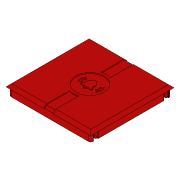
# Autodesk Inventor part: AP-03
Saved by Autodesk Inventor 2018 (Build 220112000, 112)
## iProperties
Created: 2017-11-29
Part Number: AP-03
Material: Q235
Document SubType Name: Modeling
Designer: Lars von Hebel
Mass: 170.489 g
Surface Area: 186.324 cm^2
Volume: 21.7183 cm^3
Density: 7.85 g/cm^3
Appearance: Red
RuleStatus: InUse
Author: Lars von Hebel
Autodesk Inventor part; units mm, degrees
(part 1 of 2)
ref_plane "YZ Plane" through (0, 0, 0) normal (1, 0, 0) x (0, 1, 0)
sketch "Block1" plane through (0, 0, 0) normal (0, 0, 1) x (1, 0, 0)
  spline S0 degree 3 poles (131.0781, -293.1362) (132.5466, -291.7994) (133.2816, -290.1204) (133.2816, -288.0985) (133.2816, -286.1085) (132.5466, -284.4599) (131.0781, -283.1542) knots 0 0 0 0 1 1 1 2 2 2 2
  line L0 (131.0781, -293.1362) -> (132.5466, -291.7994) construction
  line L1 (132.5466, -291.7994) -> (133.2816, -290.1204) construction
  line L2 (133.2816, -290.1204) -> (133.2816, -288.0985) construction
  line L3 (133.2816, -288.0985) -> (133.2816, -286.1085) construction
  line L4 (133.2816, -286.1085) -> (132.5466, -284.4599) construction
  line L5 (132.5466, -284.4599) -> (131.0781, -283.1542) construction
  spline S1 degree 3 poles (131.0781, -283.1542) (129.6082, -281.8485) (127.5611, -281.1953) (124.9359, -281.1953) knots 2 2 2 2 3 3 3 3
  line L6 (131.0781, -283.1542) -> (129.6082, -281.8485) construction
  line L7 (129.6082, -281.8485) -> (127.5611, -281.1953) construction
  line L8 (127.5611, -281.1953) -> (124.9359, -281.1953) construction
  line L9 (124.9359, -281.1953) -> (116.4022, -281.1953)
  line L10 (116.4022, -281.1953) -> (116.4022, -295.1414)
  line L11 (116.4022, -295.1414) -> (124.9359, -295.1414)
  spline S2 degree 3 poles (124.9359, -295.1414) (127.5611, -295.1414) (129.6082, -294.473) (131.0781, -293.1362) knots 6 6 6 6 7 7 7 7
  line L12 (124.9359, -295.1414) -> (127.5611, -295.1414) construction
  line L13 (127.5611, -295.1414) -> (129.6082, -294.473) construction
  line L14 (129.6082, -294.473) -> (131.0781, -293.1362) construction
  spline S3 degree 3 poles (135.1103, -309.0643) (133.2967, -307.7434) (130.8741, -307.0822) (127.8425, -307.0822) knots 0 0 0 0 1 1 1 1
  line L15 (135.1103, -309.0643) -> (133.2967, -307.7434) construction
  line L16 (133.2967, -307.7434) -> (130.8741, -307.0822) construction
  line L17 (130.8741, -307.0822) -> (127.8425, -307.0822) construction
  line L18 (127.8425, -307.0822) -> (116.4022, -307.0822)
  line L19 (116.4022, -307.0822) -> (116.4022, -322.4743)
  line L20 (116.4022, -322.4743) -> (125.592, -322.4743)
  spline S4 degree 3 poles (125.592, -322.4743) (129.9366, -322.4743) (133.0624, -321.876) (134.9699, -320.6788) knots 4 4 4 4 5 5 5 5
  line L21 (125.592, -322.4743) -> (129.9366, -322.4743) construction
  line L22 (129.9366, -322.4743) -> (133.0624, -321.876) construction
  line L23 (133.0624, -321.876) -> (134.9699, -320.6788) construction
  spline S5 degree 3 poles (134.9699, -320.6788) (136.876, -319.4816) (137.8294, -317.4063) (137.8294, -314.452) (137.8294, -312.182) (136.923, -310.3866) (135.1103, -309.0643) knots 5 5 5 5 6 6 6 7 7 7 7
  line L24 (134.9699, -320.6788) -> (136.876, -319.4816) construction
  line L25 (136.876, -319.4816) -> (137.8294, -317.4063) construction
  line L26 (137.8294, -317.4063) -> (137.8294, -314.452) construction
  line L27 (137.8294, -314.452) -> (137.8294, -312.182) construction
  line L28 (137.8294, -312.182) -> (136.923, -310.3866) construction
  line L29 (136.923, -310.3866) -> (135.1103, -309.0643) construction
  spline S6 degree 3 poles (123.151, -216.2055) (123.151, -206.5504) (130.9712, -198.7334) (140.6263, -198.7334) knots 0 0 0 0 1 1 1 1
  line L30 (123.151, -216.2055) -> (123.151, -206.5504) construction
  line L31 (123.151, -206.5504) -> (130.9712, -198.7334) construction
  line L32 (130.9712, -198.7334) -> (140.6263, -198.7334) construction
  line L33 (140.6263, -198.7334) -> (140.6263, -159.7323)
  spline S7 degree 3 poles (140.6263, -159.7323) (140.6263, -132.2619) (159.7288, -109.3026) (185.3549, -103.2715) knots 2 2 2 2 3 3 3 3
  line L34 (140.6263, -159.7323) -> (140.6263, -132.2619) construction
  line L35 (140.6263, -132.2619) -> (159.7288, -109.3026) construction
  line L36 (159.7288, -109.3026) -> (185.3549, -103.2715) construction
  spline S8 degree 3 poles (185.3549, -103.2715) (185.5067, -96.0755) (191.4085, -90.2514) (198.6594, -90.2514) (205.9045, -90.2514) (211.78, -96.0498) (211.9356, -103.2715) knots 3 3 3 3 4 4 4 5 5 5 5
  line L37 (185.3549, -103.2715) -> (185.5067, -96.0755) construction
  line L38 (185.5067, -96.0755) -> (191.4085, -90.2514) construction
  line L39 (191.4085, -90.2514) -> (198.6594, -90.2514) construction
  line L40 (198.6594, -90.2514) -> (205.9045, -90.2514) construction
  line L41 (205.9045, -90.2514) -> (211.78, -96.0498) construction
  line L42 (211.78, -96.0498) -> (211.9356, -103.2715) construction
  spline S9 degree 3 poles (211.9356, -103.2715) (237.5617, -109.3026) (256.6634, -132.2619) (256.6634, -159.7323) knots 5 5 5 5 6 6 6 6
  line L43 (211.9356, -103.2715) -> (237.5617, -109.3026) construction
  line L44 (237.5617, -109.3026) -> (256.6634, -132.2619) construction
  line L45 (256.6634, -132.2619) -> (256.6634, -159.7323) construction
  line L46 (256.6634, -159.7323) -> (256.6634, -198.7334)
  spline S10 degree 3 poles (256.6634, -198.7334) (266.3194, -198.7334) (274.1356, -206.5504) (274.1356, -216.2055) knots 7 7 7 7 8 8 8 8
  line L47 (256.6634, -198.7334) -> (266.3194, -198.7334) construction
  line L48 (266.3194, -198.7334) -> (274.1356, -206.5504) construction
  line L49 (274.1356, -206.5504) -> (274.1356, -216.2055) construction
  line L50 (274.1356, -216.2055) -> (274.1356, -228.533)
  line L51 (274.1356, -228.533) -> (123.151, -228.533)
  line L52 (123.151, -228.533) -> (123.151, -216.2055)
  spline S11 degree 3 poles (75.656, -215.1488) (74.5193, -215.883) (73.2455, -216.2339) (71.9859, -216.2339) (69.7638, -216.2339) (67.5867, -215.1414) (66.2906, -213.1359) (55.8364, -196.9575) (50.3107, -178.1799) (50.3107, -158.8331) (50.3107, -139.9897) (55.5725, -121.6274) (65.5276, -105.7302) (67.5128, -102.5603) (71.6917, -101.5976) (74.8633, -103.5844) (78.0341, -105.57) (78.9947, -109.7497) (77.0092, -112.92) (68.4053, -126.6596) (63.8576, -142.536) (63.8576, -158.8331) (63.8576, -175.5656) (68.6335, -191.8008) (77.6688, -205.7835) (79.699, -208.9255) (78.7979, -213.1184) (75.656, -215.1488) knots 0 0 0 0 1 1 1 2 2 2 3 3 3 4 4 4 5 5 5 6 6 6 7 7 7 8 8 8 9 9 9 9
  line L53 (75.656, -215.1488) -> (74.5193, -215.883) construction
  line L54 (74.5193, -215.883) -> (73.2455, -216.2339) construction
  line L55 (73.2455, -216.2339) -> (71.9859, -216.2339) construction
  line L56 (71.9859, -216.2339) -> (69.7638, -216.2339) construction
  line L57 (69.7638, -216.2339) -> (67.5867, -215.1414) construction
  line L58 (67.5867, -215.1414) -> (66.2906, -213.1359) construction
  line L59 (66.2906, -213.1359) -> (55.8364, -196.9575) construction
  line L60 (55.8364, -196.9575) -> (50.3107, -178.1799) construction
  line L61 (50.3107, -178.1799) -> (50.3107, -158.8331) construction
  line L62 (50.3107, -158.8331) -> (50.3107, -139.9897) construction
  line L63 (50.3107, -139.9897) -> (55.5725, -121.6274) construction
  line L64 (55.5725, -121.6274) -> (65.5276, -105.7302) construction
  line L65 (65.5276, -105.7302) -> (67.5128, -102.5603) construction
  line L66 (67.5128, -102.5603) -> (71.6917, -101.5976) construction
  line L67 (71.6917, -101.5976) -> (74.8633, -103.5844) construction
  line L68 (74.8633, -103.5844) -> (78.0341, -105.57) construction
  line L69 (78.0341, -105.57) -> (78.9947, -109.7497) construction
  line L70 (78.9947, -109.7497) -> (77.0092, -112.92) construction
  line L71 (77.0092, -112.92) -> (68.4053, -126.6596) construction
  line L72 (68.4053, -126.6596) -> (63.8576, -142.536) construction
  line L73 (63.8576, -142.536) -> (63.8576, -158.8331) construction
  line L74 (63.8576, -158.8331) -> (63.8576, -175.5656) construction
  line L75 (63.8576, -175.5656) -> (68.6335, -191.8008) construction
  line L76 (68.6335, -191.8008) -> (77.6688, -205.7835) construction
  line L77 (77.6688, -205.7835) -> (79.699, -208.9255) construction
  line L78 (79.699, -208.9255) -> (78.7979, -213.1184) construction
  line L79 (78.7979, -213.1184) -> (75.656, -215.1488) construction
  spline S12 degree 3 poles (91.7394, -196.7237) (84.4441, -185.4332) (80.5881, -172.331) (80.5881, -158.8331) (80.5881, -145.6846) (84.2605, -132.8708) (91.2083, -121.7772) (93.0767, -118.7927) (97.0101, -117.8885) (99.9949, -119.7577) (102.9789, -121.6266) (103.8828, -125.5604) (102.0143, -128.5443) (96.3382, -137.6073) (93.3382, -148.0811) (93.3382, -158.8331) (93.3382, -169.8707) (96.4884, -180.5803) (102.4482, -189.804) (104.359, -192.7611) (103.5109, -196.7078) (100.5536, -198.6182) (99.484, -199.3093) (98.2848, -199.6396) (97.0996, -199.6396) (95.0078, -199.6396) (92.9592, -198.6112) (91.7394, -196.7237) knots 0 0 0 0 1 1 1 2 2 2 3 3 3 4 4 4 5 5 5 6 6 6 7 7 7 8 8 8 9 9 9 9
  line L80 (91.7394, -196.7237) -> (84.4441, -185.4332) construction
  line L81 (84.4441, -185.4332) -> (80.5881, -172.331) construction
  line L82 (80.5881, -172.331) -> (80.5881, -158.8331) construction
  line L83 (80.5881, -158.8331) -> (80.5881, -145.6846) construction
  line L84 (80.5881, -145.6846) -> (84.2605, -132.8708) construction
  line L85 (84.2605, -132.8708) -> (91.2083, -121.7772) construction
  line L86 (91.2083, -121.7772) -> (93.0767, -118.7927) construction
  line L87 (93.0767, -118.7927) -> (97.0101, -117.8885) construction
  line L88 (97.0101, -117.8885) -> (99.9949, -119.7577) construction
  line L89 (99.9949, -119.7577) -> (102.9789, -121.6266) construction
  line L90 (102.9789, -121.6266) -> (103.8828, -125.5604) construction
  line L91 (103.8828, -125.5604) -> (102.0143, -128.5443) construction
  line L92 (102.0143, -128.5443) -> (96.3382, -137.6073) construction
  line L93 (96.3382, -137.6073) -> (93.3382, -148.0811) construction
  line L94 (93.3382, -148.0811) -> (93.3382, -158.8331) construction
  line L95 (93.3382, -158.8331) -> (93.3382, -169.8707) construction
  line L96 (93.3382, -169.8707) -> (96.4884, -180.5803) construction
  line L97 (96.4884, -180.5803) -> (102.4482, -189.804) construction
  line L98 (102.4482, -189.804) -> (104.359, -192.7611) construction
  line L99 (104.359, -192.7611) -> (103.5109, -196.7078) construction
  line L100 (103.5109, -196.7078) -> (100.5536, -198.6182) construction
  line L101 (100.5536, -198.6182) -> (99.484, -199.3093) construction
  line L102 (99.484, -199.3093) -> (98.2848, -199.6396) construction
  line L103 (98.2848, -199.6396) -> (97.0996, -199.6396) construction
  line L104 (97.0996, -199.6396) -> (95.0078, -199.6396) construction
  line L105 (95.0078, -199.6396) -> (92.9592, -198.6112) construction
  line L106 (92.9592, -198.6112) -> (91.7394, -196.7237) construction
  spline S13 degree 3 poles (149.2234, -329.0939) (145.3157, -332.6421) (139.5648, -334.4151) (131.9686, -334.4151) knots 0 0 0 0 1 1 1 1
  line L107 (149.2234, -329.0939) -> (145.3157, -332.6421) construction
  line L108 (145.3157, -332.6421) -> (139.5648, -334.4151) construction
  line L109 (139.5648, -334.4151) -> (131.9686, -334.4151) construction
  line L110 (131.9686, -334.4151) -> (100.0857, -334.4151)
  line L111 (100.0857, -334.4151) -> (100.0857, -269.2545)
  line L112 (100.0857, -269.2545) -> (128.4053, -269.2545)
  spline S14 degree 3 poles (128.4053, -269.2545) (135.1573, -269.2545) (140.4625, -270.8705) (144.3239, -274.1019) knots 4 4 4 4 5 5 5 5
  line L113 (128.4053, -269.2545) -> (135.1573, -269.2545) construction
  line L114 (135.1573, -269.2545) -> (140.4625, -270.8705) construction
  line L115 (140.4625, -270.8705) -> (144.3239, -274.1019) construction
  spline S15 degree 3 poles (144.3239, -274.1019) (148.1839, -277.3332) (150.1146, -281.1548) (150.1146, -285.5667) (150.1146, -291.2221) (147.1292, -295.5566) (141.1584, -298.5702) knots 5 5 5 5 6 6 6 7 7 7 7
  line L116 (144.3239, -274.1019) -> (148.1839, -277.3332) construction
  line L117 (148.1839, -277.3332) -> (150.1146, -281.1548) construction
  line L118 (150.1146, -281.1548) -> (150.1146, -285.5667) construction
  line L119 (150.1146, -285.5667) -> (150.1146, -291.2221) construction
  line L120 (150.1146, -291.2221) -> (147.1292, -295.5566) construction
  line L121 (147.1292, -295.5566) -> (141.1584, -298.5702) construction
  spline S16 degree 3 poles (141.1584, -298.5702) (145.66, -299.7529) (149.1062, -301.8377) (151.4977, -304.8245) knots 7 7 7 7 8 8 8 8
  line L122 (141.1584, -298.5702) -> (145.66, -299.7529) construction
  line L123 (145.66, -299.7529) -> (149.1062, -301.8377) construction
  line L124 (149.1062, -301.8377) -> (151.4977, -304.8245) construction
  spline S17 degree 3 poles (151.4977, -304.8245) (153.8885, -307.8121) (155.0842, -311.2966) (155.0842, -315.2788) (155.0842, -320.9421) (153.1304, -325.5472) (149.2234, -329.0939) knots 8 8 8 8 9 9 9 10 10 10 10
  line L125 (151.4977, -304.8245) -> (153.8885, -307.8121) construction
  line L126 (153.8885, -307.8121) -> (155.0842, -311.2966) construction
  line L127 (155.0842, -311.2966) -> (155.0842, -315.2788) construction
  line L128 (155.0842, -315.2788) -> (155.0842, -320.9421) construction
  line L129 (155.0842, -320.9421) -> (153.1304, -325.5472) construction
  line L130 (153.1304, -325.5472) -> (149.2234, -329.0939) construction
  line L131 (210.0365, -334.4151) -> (196.1114, -334.4151)
  line L132 (196.1114, -334.4151) -> (196.1114, -328.1181)
  spline S18 degree 3 poles (196.1114, -328.1181) (192.0156, -332.8757) (187.2493, -335.2549) (181.8102, -335.2549) (176.9961, -335.2549) (173.0891, -333.7778) (170.0886, -330.8235) knots 2 2 2 2 3 3 3 4 4 4 4
  line L133 (196.1114, -328.1181) -> (192.0156, -332.8757) construction
  line L134 (192.0156, -332.8757) -> (187.2493, -335.2549) construction
  line L135 (187.2493, -335.2549) -> (181.8102, -335.2549) construction
  line L136 (181.8102, -335.2549) -> (176.9961, -335.2549) construction
  line L137 (176.9961, -335.2549) -> (173.0891, -333.7778) construction
  line L138 (173.0891, -333.7778) -> (170.0886, -330.8235) construction
  spline S19 degree 3 poles (170.0886, -330.8235) (167.088, -327.87) (165.5877, -323.7807) (165.5877, -318.5564) knots 4 4 4 4 5 5 5 5
  line L139 (170.0886, -330.8235) -> (167.088, -327.87) construction
  line L140 (167.088, -327.87) -> (165.5877, -323.7807) construction
  line L141 (165.5877, -323.7807) -> (165.5877, -318.5564) construction
  line L142 (165.5877, -318.5564) -> (165.5877, -290.3837)
  line L143 (165.5877, -290.3837) -> (179.5127, -290.3837)
  line L144 (179.5127, -290.3837) -> (179.5127, -317.5878)
  spline S20 degree 3 poles (179.5127, -317.5878) (179.5127, -323.1774) (181.8413, -325.9725) (186.4991, -325.9725) (189.125, -325.9725) (191.3675, -324.9562) (193.2273, -322.922) (195.0871, -320.8879) (196.0174, -319.3898) (196.0174, -318.427) knots 8 8 8 8 9 9 9 10 10 10 11 11 11 11
  line L145 (179.5127, -317.5878) -> (179.5127, -323.1774) construction
  line L146 (179.5127, -323.1774) -> (181.8413, -325.9725) construction
  line L147 (181.8413, -325.9725) -> (186.4991, -325.9725) construction
  line L148 (186.4991, -325.9725) -> (189.125, -325.9725) construction
  line L149 (189.125, -325.9725) -> (191.3675, -324.9562) construction
  line L150 (191.3675, -324.9562) -> (193.2273, -322.922) construction
  line L151 (193.2273, -322.922) -> (195.0871, -320.8879) construction
  line L152 (195.0871, -320.8879) -> (196.0174, -319.3898) construction
  line L153 (196.0174, -319.3898) -> (196.0174, -318.427) construction
  line L154 (196.0174, -318.427) -> (196.0174, -290.3837)
  line L155 (196.0174, -290.3837) -> (210.0365, -290.3837)
  line L156 (210.0365, -290.3837) -> (210.0365, -334.4151)
  spline S21 degree 3 poles (198.6594, -257.2646) (187.0631, -257.2646) (177.3823, -249.4732) (174.3278, -238.8543) knots 0 0 0 0 1 1 1 1
  line L157 (198.6594, -257.2646) -> (187.0631, -257.2646) construction
  line L158 (187.0631, -257.2646) -> (177.3823, -249.4732) construction
  line L159 (177.3823, -249.4732) -> (174.3278, -238.8543) construction
  line L160 (174.3278, -238.8543) -> (222.9549, -238.8543)
  spline S22 degree 3 poles (222.9549, -238.8543) (219.9074, -249.4732) (210.2266, -257.2646) (198.6594, -257.2646) knots 2 2 2 2 3 3 3 3
  line L161 (222.9549, -238.8543) -> (219.9074, -249.4732) construction
  line L162 (219.9074, -249.4732) -> (210.2266, -257.2646) construction
  line L163 (210.2266, -257.2646) -> (198.6594, -257.2646) construction
  line L164 (263.066, -324.9468) -> (263.066, -334.4151)
  line L165 (263.066, -334.4151) -> (217.632, -334.4151)
  line L166 (217.632, -334.4151) -> (240.3605, -299.8527)
  line L167 (240.3605, -299.8527) -> (219.8354, -299.8527)
  line L168 (219.8354, -299.8527) -> (219.8354, -290.3837)
  line L169 (219.8354, -290.3837) -> (263.066, -290.3837)
  line L170 (263.066, -290.3837) -> (240.3924, -324.9468)
  line L171 (240.3924, -324.9468) -> (263.066, -324.9468)
  line L172 (313.0949, -324.9468) -> (313.0949, -334.4151)
  line L173 (313.0949, -334.4151) -> (267.6609, -334.4151)
  line L174 (267.6609, -334.4151) -> (290.3895, -299.8527)
  line L175 (290.3895, -299.8527) -> (269.8643, -299.8527)
  line L176 (269.8643, -299.8527) -> (269.8643, -290.3837)
  line L177 (269.8643, -290.3837) -> (313.0949, -290.3837)
  line L178 (313.0949, -290.3837) -> (290.4213, -324.9468)
  line L179 (290.4213, -324.9468) -> (313.0949, -324.9468)
  spline S23 degree 3 poles (307.939, -196.7233) (306.7188, -198.6108) (304.6691, -199.6396) (302.5773, -199.6396) (301.3928, -199.6396) (300.1944, -199.3097) (299.1251, -198.6187) (296.1664, -196.7078) (295.3182, -192.7615) (297.2295, -189.8043) (303.1889, -180.5799) (306.3391, -169.8703) (306.3391, -158.8331) (306.3391, -148.0799) (303.3383, -137.6065) (297.6622, -128.5448) (295.7944, -125.5607) (296.6972, -121.6269) (299.6808, -119.7582) (302.6644, -117.8881) (306.599, -118.7927) (308.4682, -121.7767) (315.416, -132.8692) (319.0891, -145.6835) (319.0891, -158.8331) (319.0891, -172.3302) (315.2323, -185.4328) (307.939, -196.7233) knots 0 0 0 0 1 1 1 2 2 2 3 3 3 4 4 4 5 5 5 6 6 6 7 7 7 8 8 8 9 9 9 9
  line L180 (307.939, -196.7233) -> (306.7188, -198.6108) construction
  line L181 (306.7188, -198.6108) -> (304.6691, -199.6396) construction
  line L182 (304.6691, -199.6396) -> (302.5773, -199.6396) construction
  line L183 (302.5773, -199.6396) -> (301.3928, -199.6396) construction
  line L184 (301.3928, -199.6396) -> (300.1944, -199.3097) construction
  line L185 (300.1944, -199.3097) -> (299.1251, -198.6187) construction
  line L186 (299.1251, -198.6187) -> (296.1664, -196.7078) construction
  line L187 (296.1664, -196.7078) -> (295.3182, -192.7615) construction
  line L188 (295.3182, -192.7615) -> (297.2295, -189.8043) construction
  line L189 (297.2295, -189.8043) -> (303.1889, -180.5799) construction
  line L190 (303.1889, -180.5799) -> (306.3391, -169.8703) construction
  line L191 (306.3391, -169.8703) -> (306.3391, -158.8331) construction
  line L192 (306.3391, -158.8331) -> (306.3391, -148.0799) construction
  line L193 (306.3391, -148.0799) -> (303.3383, -137.6065) construction
  line L194 (303.3383, -137.6065) -> (297.6622, -128.5448) construction
  line L195 (297.6622, -128.5448) -> (295.7944, -125.5607) construction
  line L196 (295.7944, -125.5607) -> (296.6972, -121.6269) construction
  line L197 (296.6972, -121.6269) -> (299.6808, -119.7582) construction
  line L198 (299.6808, -119.7582) -> (302.6644, -117.8881) construction
  line L199 (302.6644, -117.8881) -> (306.599, -118.7927) construction
  line L200 (306.599, -118.7927) -> (308.4682, -121.7767) construction
  line L201 (308.4682, -121.7767) -> (315.416, -132.8692) construction
  line L202 (315.416, -132.8692) -> (319.0891, -145.6835) construction
  line L203 (319.0891, -145.6835) -> (319.0891, -158.8331) construction
  line L204 (319.0891, -158.8331) -> (319.0891, -172.3302) construction
  line L205 (319.0891, -172.3302) -> (315.2323, -185.4328) construction
  line L206 (315.2323, -185.4328) -> (307.939, -196.7233) construction
  spline S24 degree 3 poles (333.3863, -213.1359) (332.0897, -215.1414) (329.9123, -216.2339) (327.6914, -216.2339) (326.4307, -216.2339) (325.1576, -215.8834) (324.0213, -215.1488) (320.879, -213.1184) (319.9778, -208.9255) (322.0074, -205.7835) (331.0438, -191.8) (335.8204, -175.5648) (335.8204, -158.8331) (335.8204, -142.5372) (331.2726, -126.6604) (322.6689, -112.92) (320.6829, -109.7493) (321.6431, -105.5696) (324.8151, -103.5844) (327.984, -101.5992) (332.1645, -102.5598) (334.1504, -105.7302) (344.1051, -121.6285) (349.3674, -139.9914) (349.3674, -158.8331) (349.3674, -178.1792) (343.8405, -196.9568) (333.3863, -213.1359) knots 0 0 0 0 1 1 1 2 2 2 3 3 3 4 4 4 5 5 5 6 6 6 7 7 7 8 8 8 9 9 9 9
  line L207 (333.3863, -213.1359) -> (332.0897, -215.1414) construction
  line L208 (332.0897, -215.1414) -> (329.9123, -216.2339) construction
  line L209 (329.9123, -216.2339) -> (327.6914, -216.2339) construction
  line L210 (327.6914, -216.2339) -> (326.4307, -216.2339) construction
  line L211 (326.4307, -216.2339) -> (325.1576, -215.8834) construction
  line L212 (325.1576, -215.8834) -> (324.0213, -215.1488) construction
  line L213 (324.0213, -215.1488) -> (320.879, -213.1184) construction
  line L214 (320.879, -213.1184) -> (319.9778, -208.9255) construction
  line L215 (319.9778, -208.9255) -> (322.0074, -205.7835) construction
  line L216 (322.0074, -205.7835) -> (331.0438, -191.8) construction
  line L217 (331.0438, -191.8) -> (335.8204, -175.5648) construction
  line L218 (335.8204, -175.5648) -> (335.8204, -158.8331) construction
  line L219 (335.8204, -158.8331) -> (335.8204, -142.5372) construction
  line L220 (335.8204, -142.5372) -> (331.2726, -126.6604) construction
  line L221 (331.2726, -126.6604) -> (322.6689, -112.92) construction
  line L222 (322.6689, -112.92) -> (320.6829, -109.7493) construction
  line L223 (320.6829, -109.7493) -> (321.6431, -105.5696) construction
  line L224 (321.6431, -105.5696) -> (324.8151, -103.5844) construction
  line L225 (324.8151, -103.5844) -> (327.984, -101.5992) construction
  line L226 (327.984, -101.5992) -> (332.1645, -102.5598) construction
  line L227 (332.1645, -102.5598) -> (334.1504, -105.7302) construction
  line L228 (334.1504, -105.7302) -> (344.1051, -121.6285) construction
  line L229 (344.1051, -121.6285) -> (349.3674, -139.9914) construction
  line L230 (349.3674, -139.9914) -> (349.3674, -158.8331) construction
  line L231 (349.3674, -158.8331) -> (349.3674, -178.1792) construction
  line L232 (349.3674, -178.1792) -> (343.8405, -196.9568) construction
  line L233 (343.8405, -196.9568) -> (333.3863, -213.1359) construction
  point P0 (186.8523, -231.4778)
sketch "Block2" plane through (0, 0, 0) normal (0, 0, 1) x (1, 0, 0)
  spline S0 degree 3 poles (199.9867, -151.4497) (199.9867, -151.7851) (200.1264, -151.9528) (200.4058, -151.9528) (200.5634, -151.9528) (200.6979, -151.8918) (200.8095, -151.7698) (200.9211, -151.6477) (200.9769, -151.5579) (200.9769, -151.5001) knots 8 8 8 8 9 9 9 10 10 10 11 11 11 11
  line L0 (199.9867, -151.4497) -> (199.9867, -151.7851) construction
  line L1 (199.9867, -151.7851) -> (200.1264, -151.9528) construction
  line L2 (200.1264, -151.9528) -> (200.4058, -151.9528) construction
  line L3 (200.4058, -151.9528) -> (200.5634, -151.9528) construction
  line L4 (200.5634, -151.9528) -> (200.6979, -151.8918) construction
  line L5 (200.6979, -151.8918) -> (200.8095, -151.7698) construction
  line L6 (200.8095, -151.7698) -> (200.9211, -151.6477) construction
  line L7 (200.9211, -151.6477) -> (200.9769, -151.5579) construction
  line L8 (200.9769, -151.5579) -> (200.9769, -151.5001) construction
  line L9 (200.9769, -151.5001) -> (200.9769, -149.8175)
  line L10 (200.9769, -149.8175) -> (201.8181, -149.8175)
  line L11 (201.8181, -149.8175) -> (201.8181, -152.4594)
  spline S1 degree 3 poles (201.1355, -147.8304) (200.4397, -147.8304) (199.8588, -147.3629) (199.6756, -146.7257) knots 0 0 0 0 1 1 1 1
  line L12 (201.1355, -147.8304) -> (200.4397, -147.8304) construction
  line L13 (200.4397, -147.8304) -> (199.8588, -147.3629) construction
  line L14 (199.8588, -147.3629) -> (199.6756, -146.7257) construction
  line L15 (199.6756, -146.7257) -> (202.5932, -146.7257)
  spline S2 degree 3 poles (202.5932, -146.7257) (202.4103, -147.3629) (201.8295, -147.8304) (201.1355, -147.8304) knots 2 2 2 2 3 3 3 3
  line L16 (202.5932, -146.7257) -> (202.4103, -147.3629) construction
  line L17 (202.4103, -147.3629) -> (201.8295, -147.8304) construction
  line L18 (201.8295, -147.8304) -> (201.1355, -147.8304) construction
  line L19 (204.9999, -151.8913) -> (204.9999, -152.4594)
  line L20 (204.9999, -152.4594) -> (202.2738, -152.4594)
  line L21 (202.2738, -152.4594) -> (203.6375, -150.3856)
  line L22 (203.6375, -150.3856) -> (202.406, -150.3856)
  line L23 (202.406, -150.3856) -> (202.406, -149.8175)
  line L24 (202.406, -149.8175) -> (204.9999, -149.8175)
  line L25 (204.9999, -149.8175) -> (203.6394, -151.8913)
  line L26 (203.6394, -151.8913) -> (204.9999, -151.8913)
  line L27 (208.0016, -151.8913) -> (208.0016, -152.4594)
  line L28 (208.0016, -152.4594) -> (205.2755, -152.4594)
  line L29 (205.2755, -152.4594) -> (206.6393, -150.3856)
  line L30 (206.6393, -150.3856) -> (205.4078, -150.3856)
  line L31 (205.4078, -150.3856) -> (205.4078, -149.8175)
  line L32 (205.4078, -149.8175) -> (208.0016, -149.8175)
  line L33 (208.0016, -149.8175) -> (206.6412, -151.8913)
  line L34 (206.6412, -151.8913) -> (208.0016, -151.8913)
  spline S3 degree 3 poles (207.6922, -144.1979) (207.619, -144.3111) (207.496, -144.3729) (207.3705, -144.3729) (207.2995, -144.3729) (207.2276, -144.3531) (207.1634, -144.3116) (206.9859, -144.1969) (206.935, -143.9602) (207.0497, -143.7827) (207.4072, -143.2293) (207.5962, -142.5867) (207.5962, -141.9245) (207.5962, -141.2793) (207.4162, -140.6509) (207.0756, -140.1072) (206.9636, -139.9281) (207.0177, -139.6921) (207.1967, -139.58) (207.3758, -139.4678) (207.6118, -139.522) (207.724, -139.7011) (208.1409, -140.3666) (208.3612, -141.1355) (208.3612, -141.9245) (208.3612, -142.7343) (208.1298, -143.5204) (207.6922, -144.1979) knots 0 0 0 0 1 1 1 2 2 2 3 3 3 4 4 4 5 5 5 6 6 6 7 7 7 8 8 8 9 9 9 9
  line L35 (207.6922, -144.1979) -> (207.619, -144.3111) construction
  line L36 (207.619, -144.3111) -> (207.496, -144.3729) construction
  line L37 (207.496, -144.3729) -> (207.3705, -144.3729) construction
  line L38 (207.3705, -144.3729) -> (207.2995, -144.3729) construction
  line L39 (207.2995, -144.3729) -> (207.2276, -144.3531) construction
  line L40 (207.2276, -144.3531) -> (207.1634, -144.3116) construction
  line L41 (207.1634, -144.3116) -> (206.9859, -144.1969) construction
  line L42 (206.9859, -144.1969) -> (206.935, -143.9602) construction
  line L43 (206.935, -143.9602) -> (207.0497, -143.7827) construction
  line L44 (207.0497, -143.7827) -> (207.4072, -143.2293) construction
  line L45 (207.4072, -143.2293) -> (207.5962, -142.5867) construction
  line L46 (207.5962, -142.5867) -> (207.5962, -141.9245) construction
  line L47 (207.5962, -141.9245) -> (207.5962, -141.2793) construction
  line L48 (207.5962, -141.2793) -> (207.4162, -140.6509) construction
  line L49 (207.4162, -140.6509) -> (207.0756, -140.1072) construction
  line L50 (207.0756, -140.1072) -> (206.9636, -139.9281) construction
  line L51 (206.9636, -139.9281) -> (207.0177, -139.6921) construction
  line L52 (207.0177, -139.6921) -> (207.1967, -139.58) construction
  line L53 (207.1967, -139.58) -> (207.3758, -139.4678) construction
  line L54 (207.3758, -139.4678) -> (207.6118, -139.522) construction
  line L55 (207.6118, -139.522) -> (207.724, -139.7011) construction
  line L56 (207.724, -139.7011) -> (208.1409, -140.3666) construction
  line L57 (208.1409, -140.3666) -> (208.3612, -141.1355) construction
  line L58 (208.3612, -141.1355) -> (208.3612, -141.9245) construction
  line L59 (208.3612, -141.9245) -> (208.3612, -142.7343) construction
  line L60 (208.3612, -142.7343) -> (208.1298, -143.5204) construction
  line L61 (208.1298, -143.5204) -> (207.6922, -144.1979) construction
  spline S4 degree 3 poles (209.2191, -145.1826) (209.1413, -145.303) (209.0106, -145.3685) (208.8774, -145.3685) (208.8017, -145.3685) (208.7253, -145.3475) (208.6572, -145.3034) (208.4686, -145.1816) (208.4146, -144.93) (208.5363, -144.7415) (209.0785, -143.9025) (209.3651, -142.9284) (209.3651, -141.9245) (209.3651, -140.9467) (209.0923, -139.9941) (208.576, -139.1697) (208.4569, -138.9794) (208.5145, -138.7287) (208.7048, -138.6095) (208.8949, -138.4904) (209.1458, -138.5481) (209.2649, -138.7383) (209.8622, -139.6922) (210.1779, -140.794) (210.1779, -141.9245) (210.1779, -143.0852) (209.8463, -144.2119) (209.2191, -145.1826) knots 0 0 0 0 1 1 1 2 2 2 3 3 3 4 4 4 5 5 5 6 6 6 7 7 7 8 8 8 9 9 9 9
  line L62 (209.2191, -145.1826) -> (209.1413, -145.303) construction
  line L63 (209.1413, -145.303) -> (209.0106, -145.3685) construction
  line L64 (209.0106, -145.3685) -> (208.8774, -145.3685) construction
  line L65 (208.8774, -145.3685) -> (208.8017, -145.3685) construction
  line L66 (208.8017, -145.3685) -> (208.7253, -145.3475) construction
  line L67 (208.7253, -145.3475) -> (208.6572, -145.3034) construction
  line L68 (208.6572, -145.3034) -> (208.4686, -145.1816) construction
  line L69 (208.4686, -145.1816) -> (208.4146, -144.93) construction
  line L70 (208.4146, -144.93) -> (208.5363, -144.7415) construction
  line L71 (208.5363, -144.7415) -> (209.0785, -143.9025) construction
  line L72 (209.0785, -143.9025) -> (209.3651, -142.9284) construction
  line L73 (209.3651, -142.9284) -> (209.3651, -141.9245) construction
  line L74 (209.3651, -141.9245) -> (209.3651, -140.9467) construction
  line L75 (209.3651, -140.9467) -> (209.0923, -139.9941) construction
  line L76 (209.0923, -139.9941) -> (208.576, -139.1697) construction
  line L77 (208.576, -139.1697) -> (208.4569, -138.9794) construction
  line L78 (208.4569, -138.9794) -> (208.5145, -138.7287) construction
  line L79 (208.5145, -138.7287) -> (208.7048, -138.6095) construction
  line L80 (208.7048, -138.6095) -> (208.8949, -138.4904) construction
  line L81 (208.8949, -138.4904) -> (209.1458, -138.5481) construction
  line L82 (209.1458, -138.5481) -> (209.2649, -138.7383) construction
  line L83 (209.2649, -138.7383) -> (209.8622, -139.6922) construction
  line L84 (209.8622, -139.6922) -> (210.1779, -140.794) construction
  line L85 (210.1779, -140.794) -> (210.1779, -141.9245) construction
  line L86 (210.1779, -141.9245) -> (210.1779, -143.0852) construction
  line L87 (210.1779, -143.0852) -> (209.8463, -144.2119) construction
  line L88 (209.8463, -144.2119) -> (209.2191, -145.1826) construction
  spline S5 degree 3 poles (197.0806, -149.9826) (197.1687, -149.9024) (197.2128, -149.8017) (197.2128, -149.6804) (197.2128, -149.561) (197.1687, -149.4621) (197.0806, -149.3837) knots 0 0 0 0 1 1 1 2 2 2 2
  line L89 (197.0806, -149.9826) -> (197.1687, -149.9024) construction
  line L90 (197.1687, -149.9024) -> (197.2128, -149.8017) construction
  line L91 (197.2128, -149.8017) -> (197.2128, -149.6804) construction
  line L92 (197.2128, -149.6804) -> (197.2128, -149.561) construction
  line L93 (197.2128, -149.561) -> (197.1687, -149.4621) construction
  line L94 (197.1687, -149.4621) -> (197.0806, -149.3837) construction
  spline S6 degree 3 poles (197.0806, -149.3837) (196.9924, -149.3054) (196.8696, -149.2662) (196.7121, -149.2662) knots 2 2 2 2 3 3 3 3
  line L95 (197.0806, -149.3837) -> (196.9924, -149.3054) construction
  line L96 (196.9924, -149.3054) -> (196.8696, -149.2662) construction
  line L97 (196.8696, -149.2662) -> (196.7121, -149.2662) construction
  line L98 (196.7121, -149.2662) -> (196.2, -149.2662)
  line L99 (196.2, -149.2662) -> (196.2, -150.103)
  line L100 (196.2, -150.103) -> (196.7121, -150.103)
  spline S7 degree 3 poles (196.7121, -150.103) (196.8696, -150.103) (196.9924, -150.0629) (197.0806, -149.9826) knots 6 6 6 6 7 7 7 7
  line L101 (196.7121, -150.103) -> (196.8696, -150.103) construction
  line L102 (196.8696, -150.103) -> (196.9924, -150.0629) construction
  line L103 (196.9924, -150.0629) -> (197.0806, -149.9826) construction
  spline S8 degree 3 poles (197.3225, -150.9383) (197.2137, -150.8591) (197.0683, -150.8194) (196.8864, -150.8194) knots 0 0 0 0 1 1 1 1
  line L104 (197.3225, -150.9383) -> (197.2137, -150.8591) construction
  line L105 (197.2137, -150.8591) -> (197.0683, -150.8194) construction
  line L106 (197.0683, -150.8194) -> (196.8864, -150.8194) construction
  line L107 (196.8864, -150.8194) -> (196.2, -150.8194)
  line L108 (196.2, -150.8194) -> (196.2, -151.7429)
  line L109 (196.2, -151.7429) -> (196.7514, -151.7429)
  spline S9 degree 3 poles (196.7514, -151.7429) (197.0121, -151.7429) (197.1996, -151.707) (197.3141, -151.6352) knots 4 4 4 4 5 5 5 5
  line L110 (196.7514, -151.7429) -> (197.0121, -151.7429) construction
  line L111 (197.0121, -151.7429) -> (197.1996, -151.707) construction
  line L112 (197.1996, -151.707) -> (197.3141, -151.6352) construction
  spline S10 degree 3 poles (197.3141, -151.6352) (197.4285, -151.5634) (197.4857, -151.4389) (197.4857, -151.2616) (197.4857, -151.1254) (197.4313, -151.0177) (197.3225, -150.9383) knots 5 5 5 5 6 6 6 7 7 7 7
  line L113 (197.3141, -151.6352) -> (197.4285, -151.5634) construction
  line L114 (197.4285, -151.5634) -> (197.4857, -151.4389) construction
  line L115 (197.4857, -151.4389) -> (197.4857, -151.2616) construction
  line L116 (197.4857, -151.2616) -> (197.4857, -151.1254) construction
  line L117 (197.4857, -151.1254) -> (197.4313, -151.0177) construction
  line L118 (197.4313, -151.0177) -> (197.3225, -150.9383) construction
  spline S11 degree 3 poles (196.605, -145.3668) (196.605, -144.7875) (197.0742, -144.3185) (197.6535, -144.3185) knots 0 0 0 0 1 1 1 1
  line L119 (196.605, -145.3668) -> (196.605, -144.7875) construction
  line L120 (196.605, -144.7875) -> (197.0742, -144.3185) construction
  line L121 (197.0742, -144.3185) -> (197.6535, -144.3185) construction
  line L122 (197.6535, -144.3185) -> (197.6535, -141.9784)
  spline S12 degree 3 poles (197.6535, -141.9784) (197.6535, -140.3302) (198.7996, -138.9526) (200.3372, -138.5908) knots 2 2 2 2 3 3 3 3
  line L123 (197.6535, -141.9784) -> (197.6535, -140.3302) construction
  line L124 (197.6535, -140.3302) -> (198.7996, -138.9526) construction
  line L125 (198.7996, -138.9526) -> (200.3372, -138.5908) construction
  spline S13 degree 3 poles (200.3372, -138.5908) (200.3463, -138.159) (200.7004, -137.8096) (201.5702, -137.8096) (201.9227, -138.1575) (201.932, -138.5908) knots 0 0 0 0 1 2 3 3 3 3
  line L126 (200.3372, -138.5908) -> (200.3463, -138.159) construction
  line L127 (200.3463, -138.159) -> (200.7004, -137.8096) construction
  line L128 (200.7004, -137.8096) -> (201.5702, -137.8096) construction
  line L129 (201.5702, -137.8096) -> (201.9227, -138.1575) construction
  line L130 (201.9227, -138.1575) -> (201.932, -138.5908) construction
  spline S14 degree 3 poles (201.932, -138.5908) (203.4696, -138.9526) (204.6157, -140.3302) (204.6157, -141.9784) knots 5 5 5 5 6 6 6 6
  line L131 (201.932, -138.5908) -> (203.4696, -138.9526) construction
  line L132 (203.4696, -138.9526) -> (204.6157, -140.3302) construction
  line L133 (204.6157, -140.3302) -> (204.6157, -141.9784) construction
  line L134 (204.6157, -141.9784) -> (204.6157, -144.3185)
  spline S15 degree 3 poles (204.6157, -144.3185) (205.1951, -144.3185) (205.664, -144.7875) (205.664, -145.3668) knots 7 7 7 7 8 8 8 8
  line L135 (204.6157, -144.3185) -> (205.1951, -144.3185) construction
  line L136 (205.1951, -144.3185) -> (205.664, -144.7875) construction
  line L137 (205.664, -144.7875) -> (205.664, -145.3668) construction
  line L138 (205.664, -145.3668) -> (205.664, -146.1065)
  line L139 (205.664, -146.1065) -> (196.605, -146.1065)
  line L140 (196.605, -146.1065) -> (196.605, -145.3668)
  spline S16 degree 3 poles (193.7553, -145.3034) (193.6871, -145.3475) (193.6106, -145.3685) (193.535, -145.3685) (193.4017, -145.3685) (193.2711, -145.303) (193.1933, -145.1826) (192.5661, -144.2119) (192.2345, -143.0853) (192.2345, -141.9245) (192.2345, -140.7939) (192.5502, -139.6921) (193.1476, -138.7383) (193.2667, -138.5481) (193.5174, -138.4903) (193.7077, -138.6095) (193.8979, -138.7287) (193.9556, -138.9795) (193.8364, -139.1697) (193.3202, -139.994) (193.0474, -140.9466) (193.0474, -141.9245) (193.0474, -142.9284) (193.3339, -143.9025) (193.876, -144.7415) (193.9978, -144.93) (193.9438, -145.1816) (193.7553, -145.3034) knots 0 0 0 0 1 1 1 2 2 2 3 3 3 4 4 4 5 5 5 6 6 6 7 7 7 8 8 8 9 9 9 9
  line L141 (193.7553, -145.3034) -> (193.6871, -145.3475) construction
  line L142 (193.6871, -145.3475) -> (193.6106, -145.3685) construction
  line L143 (193.6106, -145.3685) -> (193.535, -145.3685) construction
  line L144 (193.535, -145.3685) -> (193.4017, -145.3685) construction
  line L145 (193.4017, -145.3685) -> (193.2711, -145.303) construction
  line L146 (193.2711, -145.303) -> (193.1933, -145.1826) construction
  line L147 (193.1933, -145.1826) -> (192.5661, -144.2119) construction
  line L148 (192.5661, -144.2119) -> (192.2345, -143.0853) construction
  line L149 (192.2345, -143.0853) -> (192.2345, -141.9245) construction
  line L150 (192.2345, -141.9245) -> (192.2345, -140.7939) construction
  line L151 (192.2345, -140.7939) -> (192.5502, -139.6921) construction
  line L152 (192.5502, -139.6921) -> (193.1476, -138.7383) construction
  line L153 (193.1476, -138.7383) -> (193.2667, -138.5481) construction
  line L154 (193.2667, -138.5481) -> (193.5174, -138.4903) construction
  line L155 (193.5174, -138.4903) -> (193.7077, -138.6095) construction
  line L156 (193.7077, -138.6095) -> (193.8979, -138.7287) construction
  line L157 (193.8979, -138.7287) -> (193.9556, -138.9795) construction
  line L158 (193.9556, -138.9795) -> (193.8364, -139.1697) construction
  line L159 (193.8364, -139.1697) -> (193.3202, -139.994) construction
  line L160 (193.3202, -139.994) -> (193.0474, -140.9466) construction
  line L161 (193.0474, -140.9466) -> (193.0474, -141.9245) construction
  line L162 (193.0474, -141.9245) -> (193.0474, -142.9284) construction
  line L163 (193.0474, -142.9284) -> (193.3339, -143.9025) construction
  line L164 (193.3339, -143.9025) -> (193.876, -144.7415) construction
  line L165 (193.876, -144.7415) -> (193.9978, -144.93) construction
  line L166 (193.9978, -144.93) -> (193.9438, -145.1816) construction
  line L167 (193.9438, -145.1816) -> (193.7553, -145.3034) construction
  spline S17 degree 3 poles (194.7203, -144.1979) (194.2825, -143.5205) (194.0512, -142.7343) (194.0512, -141.9245) (194.0512, -141.1356) (194.2715, -140.3667) (194.6884, -139.7011) (194.8005, -139.522) (195.0365, -139.4678) (195.2156, -139.5799) (195.3946, -139.6921) (195.4489, -139.9281) (195.3368, -140.1071) (194.9962, -140.6509) (194.8162, -141.2793) (194.8162, -141.9245) (194.8162, -142.5867) (195.0052, -143.2293) (195.3628, -143.7827) (195.4774, -143.9601) (195.4265, -144.1969) (195.2491, -144.3116) (195.1849, -144.353) (195.113, -144.3729) (195.0419, -144.3729) (194.9164, -144.3729) (194.7934, -144.3111) (194.7203, -144.1979) knots 0 0 0 0 1 1 1 2 2 2 3 3 3 4 4 4 5 5 5 6 6 6 7 7 7 8 8 8 9 9 9 9
  line L168 (194.7203, -144.1979) -> (194.2825, -143.5205) construction
  line L169 (194.2825, -143.5205) -> (194.0512, -142.7343) construction
  line L170 (194.0512, -142.7343) -> (194.0512, -141.9245) construction
  line L171 (194.0512, -141.9245) -> (194.0512, -141.1356) construction
  line L172 (194.0512, -141.1356) -> (194.2715, -140.3667) construction
  line L173 (194.2715, -140.3667) -> (194.6884, -139.7011) construction
  line L174 (194.6884, -139.7011) -> (194.8005, -139.522) construction
  line L175 (194.8005, -139.522) -> (195.0365, -139.4678) construction
  line L176 (195.0365, -139.4678) -> (195.2156, -139.5799) construction
  line L177 (195.2156, -139.5799) -> (195.3946, -139.6921) construction
  line L178 (195.3946, -139.6921) -> (195.4489, -139.9281) construction
  line L179 (195.4489, -139.9281) -> (195.3368, -140.1071) construction
  line L180 (195.3368, -140.1071) -> (194.9962, -140.6509) construction
  line L181 (194.9962, -140.6509) -> (194.8162, -141.2793) construction
  line L182 (194.8162, -141.2793) -> (194.8162, -141.9245) construction
  line L183 (194.8162, -141.9245) -> (194.8162, -142.5867) construction
  line L184 (194.8162, -142.5867) -> (195.0052, -143.2293) construction
  line L185 (195.0052, -143.2293) -> (195.3628, -143.7827) construction
  line L186 (195.3628, -143.7827) -> (195.4774, -143.9601) construction
  line L187 (195.4774, -143.9601) -> (195.4265, -144.1969) construction
  line L188 (195.4265, -144.1969) -> (195.2491, -144.3116) construction
  line L189 (195.2491, -144.3116) -> (195.1849, -144.353) construction
  line L190 (195.1849, -144.353) -> (195.113, -144.3729) construction
  line L191 (195.113, -144.3729) -> (195.0419, -144.3729) construction
  line L192 (195.0419, -144.3729) -> (194.9164, -144.3729) construction
  line L193 (194.9164, -144.3729) -> (194.7934, -144.3111) construction
  line L194 (194.7934, -144.3111) -> (194.7203, -144.1979) construction
  spline S18 degree 3 poles (198.1693, -152.1401) (197.9348, -152.353) (197.5898, -152.4594) (197.134, -152.4594) knots 0 0 0 0 1 1 1 1
  line L195 (198.1693, -152.1401) -> (197.9348, -152.353) construction
  line L196 (197.9348, -152.353) -> (197.5898, -152.4594) construction
  line L197 (197.5898, -152.4594) -> (197.134, -152.4594) construction
  line L198 (197.134, -152.4594) -> (195.221, -152.4594)
  line L199 (195.221, -152.4594) -> (195.221, -148.5497)
  line L200 (195.221, -148.5497) -> (196.9202, -148.5497)
  spline S19 degree 3 poles (196.9202, -148.5497) (197.3253, -148.5497) (197.6436, -148.6467) (197.8753, -148.8406) knots 4 4 4 4 5 5 5 5
  line L201 (196.9202, -148.5497) -> (197.3253, -148.5497) construction
  line L202 (197.3253, -148.5497) -> (197.6436, -148.6467) construction
  line L203 (197.6436, -148.6467) -> (197.8753, -148.8406) construction
  spline S20 degree 3 poles (197.8753, -148.8406) (198.1069, -149.0345) (198.2228, -149.2638) (198.2228, -149.5285) (198.2228, -149.8678) (198.0436, -150.1279) (197.6854, -150.3087) knots 5 5 5 5 6 6 6 7 7 7 7
  line L204 (197.8753, -148.8406) -> (198.1069, -149.0345) construction
  line L205 (198.1069, -149.0345) -> (198.2228, -149.2638) construction
  line L206 (198.2228, -149.2638) -> (198.2228, -149.5285) construction
  line L207 (198.2228, -149.5285) -> (198.2228, -149.8678) construction
  line L208 (198.2228, -149.8678) -> (198.0436, -150.1279) construction
  line L209 (198.0436, -150.1279) -> (197.6854, -150.3087) construction
  spline S21 degree 3 poles (197.6854, -150.3087) (197.9555, -150.3797) (198.1623, -150.5047) (198.3058, -150.6839) knots 7 7 7 7 8 8 8 8
  line L210 (197.6854, -150.3087) -> (197.9555, -150.3797) construction
  line L211 (197.9555, -150.3797) -> (198.1623, -150.5047) construction
  line L212 (198.1623, -150.5047) -> (198.3058, -150.6839) construction
  spline S22 degree 3 poles (198.3058, -150.6839) (198.4492, -150.8632) (198.5209, -151.0723) (198.5209, -151.3112) (198.5209, -151.651) (198.4037, -151.9273) (198.1693, -152.1401) knots 8 8 8 8 9 9 9 10 10 10 10
  line L213 (198.3058, -150.6839) -> (198.4492, -150.8632) construction
  line L214 (198.4492, -150.8632) -> (198.5209, -151.0723) construction
  line L215 (198.5209, -151.0723) -> (198.5209, -151.3112) construction
  line L216 (198.5209, -151.3112) -> (198.5209, -151.651) construction
  line L217 (198.5209, -151.651) -> (198.4037, -151.9273) construction
  line L218 (198.4037, -151.9273) -> (198.1693, -152.1401) construction
  line L219 (201.8181, -152.4594) -> (200.9826, -152.4594)
  line L220 (200.9826, -152.4594) -> (200.9826, -152.0816)
  spline S23 degree 3 poles (200.9826, -152.0816) (200.7368, -152.367) (200.4509, -152.5098) (200.1245, -152.5098) (199.8357, -152.5098) (199.6012, -152.4211) (199.4212, -152.2439) knots 2 2 2 2 3 3 3 4 4 4 4
  line L221 (200.9826, -152.0816) -> (200.7368, -152.367) construction
  line L222 (200.7368, -152.367) -> (200.4509, -152.5098) construction
  line L223 (200.4509, -152.5098) -> (200.1245, -152.5098) construction
  line L224 (200.1245, -152.5098) -> (199.8357, -152.5098) construction
  line L225 (199.8357, -152.5098) -> (199.6012, -152.4211) construction
  line L226 (199.6012, -152.4211) -> (199.4212, -152.2439) construction
  spline S24 degree 3 poles (199.4212, -152.2439) (199.2412, -152.0667) (199.1512, -151.8213) (199.1512, -151.5079) knots 4 4 4 4 5 5 5 5
  line L227 (199.4212, -152.2439) -> (199.2412, -152.0667) construction
  line L228 (199.2412, -152.0667) -> (199.1512, -151.8213) construction
  line L229 (199.1512, -151.8213) -> (199.1512, -151.5079) construction
  line L230 (199.1512, -151.5079) -> (199.1512, -149.8175)
  line L231 (199.1512, -149.8175) -> (199.9867, -149.8175)
  line L232 (199.9867, -149.8175) -> (199.9867, -151.4497)
  point P0 (200.4244, -146.3146)